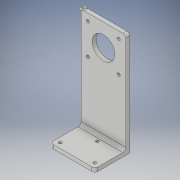
# Autodesk Inventor part: Suporte Esquerdo 2
Saved by Autodesk Inventor 2017 (Build 210142000, 142)
## iProperties
Created: 2016-09-25
Part Number: Suporte Esquerdo 2
Material: Generic
Document SubType Name: Modeling
Designer: mateu
Density: 1 g/cm^3
Appearance: Default
Author: mateu
Autodesk Inventor part; units mm, degrees
ref_plane "YZ Plane" through (0, 0, 0) normal (1, 0, 0) x (0, 1, 0)
ref_plane "XZ Plane" through (0, 0, 0) normal (0, 1, 0) x (-1, 0, 0)
ref_plane "XY Plane" through (0, 0, 0) normal (0, 0, 1) x (1, 0, 0)
sketch "Sketch1" plane through (0, 0, 0) normal (0, 0, 1) x (1, 0, 0)
  point P0 (0, 0)
sketch "Sketch2" plane through (0, 0, 0) normal (0, 0, 1) x (1, 0, 0)
  line L0 (0, 0) -> (45, 0)
  line L1 (45, 0) -> (45, -105)
  line L2 (45, -105) -> (0, -105)
  line L3 (0, -105) -> (0, 0)
  circle A0 centre (7, -7) radius 1.5
  circle A1 centre (7, -38) radius 1.5
  circle A2 centre (38, -7) radius 1.5
  circle A3 centre (38, -38) radius 1.5
  circle A4 centre (22.5, -22.5) radius 11.5
  dimension "d0" = 45
  dimension "d1" = 105
  dimension "d2" = 3
  dimension "d3" = 3
  dimension "d4" = 3
  dimension "d5" = 3
  dimension "d6" = 31
  dimension "d10" = 7
  dimension "d11" = 7
  dimension "d12" = 31
  dimension "d13" = 7
  dimension "d14" = 7
  dimension "d15" = 31
  dimension "d16" = 31
  dimension "d17" = 23
  dimension "d18" = 22.5
  dimension "d19" = 22.5
  constraints: 8 end point, 5 centre point, 2 parallel, 1 horizontal, 1 perpendicular
  measures "d0" distance of L1.end L2.end
  measures "d1" distance of L0.end L1.end
  measures "d2" diameter of A0
  measures "d3" diameter of A1
  measures "d4" diameter of A2
  measures "d5" diameter of A3
  measures "d6" distance of A2.centre A0.centre
  measures "d10" distance from line of L3 A0.centre
  measures "d11" distance from line of L0 A0.centre
  measures "d12" distance of A1.centre A0.centre
  measures "d13" distance from line of L3 A1.centre
  measures "d14" distance from line of L0 A2.centre
  measures "d15" distance of A3.centre A2.centre
  measures "d16" distance of A1.centre A3.centre
  measures "d17" diameter of A4
  measures "d18" distance from line of L3 A4.centre
  measures "d19" distance from line of L0 A4.centre
extrude "Extrusion1" add sketch "Sketch2" along normal blind 4
sketch "Sketch3" plane through (0, 0, 4) normal (0, 0, 1) x (1, 0, 0)
  point P0 (0, 0)
sketch "Sketch4" plane through (0, 0, 4) normal (0, 0, 1) x (1, 0, 0)
  line L0 (0, 0) -> (0, -105) projected
  line L1 (45, -105) -> (45, 0) projected
  line L2 (0, 0) -> (45, 0)
  line L3 (45, 0) -> (45, -105)
  line L4 (45, -105) -> (0, -105)
  line L5 (0, -105) -> (0, 0)
  line L6 (0, -105) -> (45, -105)
  line L7 (45, -105) -> (45, -101)
  line L8 (45, -101) -> (0, -101)
  line L9 (0, -101) -> (0, -105)
  dimension "d22" = 4
  constraints: 16 end point, 4 parallel, 2 horizontal, 2 perpendicular, 1 point on line
  measures "d22" distance of L7.end L6.end
extrude "Extrusion2" add sketch "Sketch4" along normal blind 31 contours L8 L1 L4 L0
sketch "Sketch5" plane through (0, -101, 4) normal (0, 1, 0) x (1, 0, 0)
  line L0 (45, 4) -> (0, 4) projected
  line L1 (45, 4) -> (45, -31) projected
  line L2 (0, 4) -> (45, 4)
  line L3 (45, 4) -> (45, -31)
  line L4 (45, -31) -> (0, -31)
  line L5 (0, -31) -> (0, 4)
  circle A0 centre (5, -26) radius 1.5
  circle A1 centre (40, -26) radius 1.5
  circle A2 centre (22.5, -6) radius 1.5
  dimension "d25" = 3
  dimension "d26" = 3
  dimension "d27" = 3
  dimension "d28" = 5
  dimension "d29" = 5
  dimension "d30" = 5
  dimension "d31" = 5
  dimension "d32" = 22.5
  dimension "d33" = 25
  constraints: 8 end point, 3 centre point, 2 parallel, 1 horizontal, 1 perpendicular
  measures "d25" diameter of A0
  measures "d26" diameter of A1
  measures "d27" diameter of A2
  measures "d28" distance from line of L5 A0.centre
  measures "d29" distance from line of L4 A0.centre
  measures "d30" distance from line of L1 A1.centre
  measures "d31" distance from line of L4 A1.centre
  measures "d32" distance from line of L5 A2.centre
  measures "d33" distance from line of L4 A2.centre
extrude "Extrusion3" cut sketch "Sketch5" against normal blind 4 contours A0 | A1 | A2
fillet "Fillet1" radius 3 1 edges at (22.5, -101, 4)
fillet "Fillet2" radius 3 1 edges at (0, 0, 2)
fillet "Fillet3" radius 3 1 edges at (0, -103, 35)
fillet "Fillet4" radius 3 1 edges at (45, -103, 35)
fillet "Fillet5" radius 3 1 edges at (45, 0, 2)
body "Solid1"
